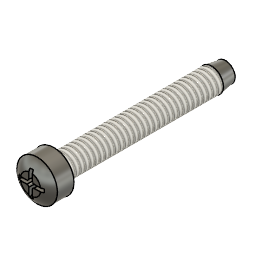
modelo_completo_v3 (Autodesk Fusion 360 archive; units mm, degrees)
design "Tornillo autorroscante taladrado con hueco cruciforme de tipo I ANSI B18.6.4 1/4-20 UNC x 1.75 Tipo C Acero grado 2 Normal"
description: Tornillo autorroscante taladrado con hueco cruciforme de tipo I ANSI B18.6.4 1/4-20 UNC x 1.75 Tipo C
part number: CRFHTSTCTI ANSI B18.6.4 - 1/4 - 20 x 1 3/4 Acero grado 2 Normal
Autodesk Fusion 360 part; units mm, degrees
note: some values were not read from the file. Chosen so that the rebuilt part matches the saved one: which bodies a step acts on; which face or edge a step refers to; how an offset face is resized; the sign of a taper; which pieces of a blend or face edit are solid. Set by a fixed rule: which sketch regions a step uses.
sketch "Sketch1" plane through (0, 0, 0) normal (0, 1, 0) x (1, 0, 0)
  line L0 (-3.175, 0) -> (-3.175, 44.45)
  line L1 (-3.175, 44.45) -> (0, 44.45)
  line L2 (0, 44.45) -> (0, -6.0198)
  line L3 (-3.175, 0) -> (-5.2578, 0)
  line L4 (-5.2578, 0) -> (-5.2578, -4.318)
  arc A0 (-5.2578, -4.318) -> (-2.6289, -6.0198) centre (0, 0.9227) ccw
  line L5 (0, -6.0198) -> (-2.6289, -6.0198)
  dimension "d9" = 6.35
  dimension "d66" = 10.5156
  dimension "d122" = 6.0198
  dimension "d123" = 1.7018
  dimension "d124" = 5.2578
  dimension "d125" = 44.45
  constraint perpendicular L0 L1
  constraint perpendicular L0 L3
  constraint coincident origin L3
  constraint vertical L0
  constraint vertical L2
  constraint coincident L2 A0.centre
  constraint coincident origin L2
  constraint vertical L4
  constraint perpendicular L2 L5
  constraint coincident L2 L5.start
  constraint coincident L2.end L5.start
  measures "d122" distance of L3 L5
  measures "d123" distance of L4.end L5
  measures "d125" distance of origin L1
revolve "Revolve1" add sketch "Sketch1" angle 360 about axis through (0, 0, -44.45) along (0, 0, 1) makes body 1
ref_plane "WorkPlane1" through (0, 0, 6.0198) normal (0, 0, 1) x (1, 0, 0)
sketch "Sketch2" plane through (0, 0, 6.0198) normal (0, 0, 1) x (1, 0, 0)
  line L0 (-0.4572, -0.4572) -> (-3.4798, -0.4572)
  line L1 (-3.4798, 0.4572) -> (-0.4572, 0.4572)
  line L2 (-3.4798, -0.4572) -> (-3.4798, 0.4572)
  line L3 (-0.4572, -3.4798) -> (-0.4572, -0.4572)
  line L4 (0.4572, -3.4798) -> (-0.4572, -3.4798)
  line L5 (0.4572, -0.4572) -> (0.4572, -3.4798)
  line L6 (3.4798, -0.4572) -> (0.4572, -0.4572)
  line L7 (3.4798, 0.4572) -> (3.4798, -0.4572)
  line L8 (0.4572, 0.4572) -> (3.4798, 0.4572)
  line L9 (0.4572, 3.4798) -> (0.4572, 0.4572)
  line L10 (-0.4572, 3.4798) -> (0.4572, 3.4798)
  line L11 (-0.4572, 0.4572) -> (-0.4572, 3.4798)
  circle A0 centre (0, 0) radius 3.4798 construction
  dimension "d132" = 360
  dimension "d138" = 0.9144
  dimension "d139" = 6.9596
  constraint coincident A0.centre origin
  constraint coincident L0.end L2.start
  constraint horizontal L1
  constraint vertical L0.start L1.end
  constraint coincident L1.end L11.start
  constraint perpendicular L1 L2
  constraint tangent L10 A0
  measures "d138" distance of L0 L1
  measures "d139" diameter of A0
extrude "Extrude2" add sketch "Sketch2" against normal blind 3.7592 draft -4 separate body makes body 2
draft "Draft2" angle -30 neutral plane through (0, 0, 6.0198) pull (0, 0, 1) 4 faces at (-3.3922, 0.0648, 4.7667) (0.0648, -3.3922, 4.7667) (3.3922, 0.0648, 4.7667) (0.0648, 3.3922, 4.7667) on bodies 2
fillet "Fillet4" radius 0.4572 4 edges at (-0.3258, 0.3258, 4.1402) (0.3258, 0.3258, 4.1402) (-0.3258, -0.3258, 4.1402) (0.3258, -0.3258, 4.1402) on bodies 2
combine "Combine1" operation cut target body 1 tool bodies 2
thread "Thread1" "ANSI Unified Screw Threads 0.25 1/4-20 UNC 1/4-20 UNC 2A" major diameter 6.2205 minor diameter 4.8108 pitch 1.27 angle 60 resizes the face on face at (-3.1711, 0.1583, -14.8167) on bodies 1
sketch "Sketch5" plane through (0, 0, 0) normal (0, 1, 0) x (1, 0, 0)
  line L0 (-3.2385, 40.005) -> (-2.54, 44.45)
  line L1 (-3.2385, 40.005) -> (-3.2385, 44.45)
  line L2 (0, 44.45) -> (0, -6.0198)
  line L3 (-3.2385, 44.45) -> (0, 44.45)
  dimension "d126" = 0.6985
  dimension "d127" = 3.2385
  dimension "d128" = 4.445
  constraint coincident L2.start L3.end
  constraint perpendicular L2 L3
  constraint coincident L0.end L3
  constraint perpendicular L1 L3
  measures "d126" distance of L0.end L1
  measures "d127" distance of L1 L2.start
  measures "d128" distance of L0.start L3
revolve "Revolve2" cut sketch "Sketch5" angle 360 about axis through (0, 0, -44.45) along (0, 0, 1) bodies 1
equation "d9 = adsk_nomdia"
equation "d66 = adsk_headdia"
equation "d71 = adsk_headh"
equation "adsk_nomlen = 1.75 in"
equation "adsk_headh = 0.237 in"
equation "adsk_headdia = 0.414 in"
equation "adsk_nomdia = 0.25 in"
equation "adsk_phildia = 0.274 in"
equation "adsk_philwidth = 0.036 in"
equation "adsk_phildepth = 0.148 in"
equation "adsk_startlen = 0.175 in"
equation "adsk_endpointdia = 0.20 in"
equation "d111 = -adsk_phildepth"
equation "adsk_ovalh = 0.067 in"
equation "d122 = adsk_headh"
equation "d123 = adsk_ovalh"
equation "d124 = adsk_headdia * 0.5"
equation "d125 = adsk_nomlen"
equation "d126 = ( 0.51 * adsk_nomdia ) - ( adsk_endpointdia / 2 )"
equation "d127 = 0.51 * adsk_nomdia"
equation "d128 = adsk_startlen"
equation "d136 = adsk_philwidth / 2"
equation "d138 = adsk_philwidth"
equation "d139 = adsk_phildia"

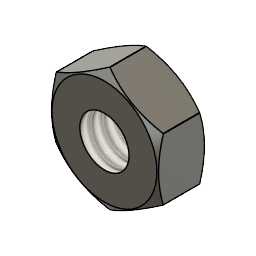
design "Tuerca para maquinaria hexagonal perfil bajo achaflanada ASME B18.6.3 - 1/4-20 Acero grado 2H Normal"
description: Tuerca para maquinaria hexagonal perfil bajo achaflanada ASME B18.6.3 - 1/4-20
part number: CBHMSN ASME B18.6.3 - 1/4-20 Acero grado 2H Normal
Autodesk Fusion 360 part; units mm, degrees
sketch "Sketch1" plane through (0, 0, 0) normal (0, 1, 0) x (1, 0, 0)
  line L0 (0, 0) -> (0, -4.9022)
  line L1 (-3.175, 0) -> (-5.4513, 0)
  line L2 (-5.4513, 0) -> (-6.4135, -0.5555)
  line L3 (-6.4135, -0.5555) -> (-6.4135, -4.3467)
  line L4 (-6.4135, -4.3467) -> (-5.4513, -4.9022)
  line L5 (-5.4513, -4.9022) -> (-3.175, -4.9022)
  line L6 (-3.175, -4.9022) -> (-3.175, 0)
  dimension "d121" = 6.35
  dimension "d122" = 30
  dimension "d123" = 30
  dimension "d128" = 12.827
  dimension "d142" = 10.9027
  dimension "d146" = 4.9022
  constraint vertical L0
  constraint coincident L0 L0.end
  constraint coincident origin L0
  constraint horizontal L1
  constraint coincident L0.start L1
  constraint coincident L0.start origin
  constraint vertical L1.end L4.end
  constraint coincident L0.end L5
  measures "d122" angle of L1 L2
  measures "d123" angle of L4 L5
  measures "d146" distance of L1 L5
revolve "Revolve1" add sketch "Sketch1" angle 360 about axis through (0, 0, 0) along (0, 0, 1)
sketch "Sketch8" plane through (0, 0, 4.9022) normal (0, 0, 1) x (1, 0, 0)
  line L0 (-5.5626, -3.1923) -> (-5.5626, 3.1923)
  circle A0 centre (0, 0) radius 3.175
  circle A1 centre (0, 0) radius 6.4135
  dimension "d114" = 5.5626
  constraint coincident L0.end A1
  constraint coincident L0.start A1
  constraint vertical L0
  measures "d114" distance of A0.centre L0
extrude "Extrude5" cut sketch "Sketch8" against normal blind 4.9022 contours L0 A1 picked at (-5.6999, -0.7773)
pattern_circular "C-Pattern2" count 6 over 360 about axis through (0, 0, 1.75) along (0, 0, 1) of "Extrude5"
thread "Thread3" "ANSI Unified Screw Threads 0.25 1/4-20 UNC 1/4-20 UNC 2B" major diameter 6.35 minor diameter 5.1181 pitch 1.27 angle 60 resizes the face on face at (-3.1711, 0.1583, 3.2681)
equation "d89 = -adsk_nheig"
equation "d114 = adsk_waflat / 2"
equation "adsk_chamang1 = 30 deg"
equation "adsk_chamang2 = 30 deg"
equation "d121 = adsk_nomdia"
equation "d122 = adsk_chamang1"
equation "d123 = adsk_chamang2"
equation "d128 = adsk_maxdia"
equation "adsk_nheig = 0.193 in"
equation "adsk_maxdia = 0.505 in"
equation "adsk_nomdia = 0.25 in"
equation "adsk_waflat = 0.438 in"
equation "d139 = adsk_nheig"
equation "adsk_beardia = adsk_waflat * 0.98"
equation "d142 = adsk_beardia"
equation "d146 = adsk_nheig"

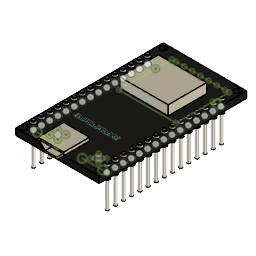
design "PINS"
part number: 2026-06-24-16-48-10-283
Autodesk Fusion 360 part; units mm, degrees
sketch "Boceto1" plane through (0, 0, 0) normal (0, 0, 1) x (1, 0, 0)
  circle A0 centre (-12.7, 17.8) radius 0.5
extrude "Extruir1" add sketch "Boceto1" along normal blind 2.5 and the other way blind 0 makes body 1
sketch "Boceto2" plane through (0, 0, 0) normal (0, 0, 1) x (1, 0, 0)
  line L0 (-14, 24) -> (12, 24)
  line L1 (12, 24) -> (12, -20)
  line L2 (12, -20) -> (-14, -20)
  line L3 (-14, -20) -> (-14, 24)
  constraint horizontal L0
  constraint vertical L1
  constraint horizontal L2
  constraint vertical L3
extrude "Extruir2" add sketch "Boceto2" along normal blind 2 separate body makes body 2
extrude "Extruir3" add 1 faces at (-12.8082, 17.6557, 0) along direction (0, 0, -1) blind 10 on bodies 1 bodies 1 2
extrude "Extruir4" add 1 faces at (3.3333, -20, 0.6667) along direction (0, -1, 0) blind 2 on bodies 1 bodies 1
sketch "Boceto3" plane through (0, 0, 2) normal (0, 0, 1) x (-1, 0, 0)
  line L0 (-12, 22) -> (-12, -24)
  line L1 (-12, -24) -> (14, -24)
  line L2 (14, -24) -> (14, 22)
  line L3 (14, 22) -> (-12, 22)
  circle A0 centre (12.7, -17.8) radius 0.5
  line L4 (12.5, -22.5) -> (12.5, 20.5)
  line L5 (12.5, 20.5) -> (-10.5, 20.5)
  line L6 (-10.5, 20.5) -> (-10.5, -22.5)
  line L7 (-10.5, -22.5) -> (12.5, -22.5)
  dimension "d11" = -1.5
hole "Agujero1" at (-12.5, 22.5, 2) at (10.5, 22.5, 2) at (-12.5, -20.5, 2) at (10.5, -20.5, 2) direction (0, 0, -1) diameter 2 depth 11 tip angle 118 bodies 1
extrude "Extruir5" add 1 faces at (-12.8082, 17.6557, 2.5) along direction (0, 0, 1) blind 0.1 on bodies 1 bodies 1
sketch "Boceto4" plane through (0, 0, 0) normal (0, 0, 1) x (1, 0, 0)
  circle A0 centre (-12.7, 17.8) radius 0.8062
extrude "Extruir6" add sketch "Boceto4" against normal blind 1.5 separate body makes body 3
sketch "Boceto5" plane through (0, 0, 2) normal (0, 0, 1) x (-1, 0, 0)
  circle A0 centre (12.7, -17.8) radius 0.5
  line L0 (-12, 22) -> (-12, -24)
  line L1 (-12, -24) -> (14, -24)
  line L2 (14, -24) -> (14, 22)
  line L3 (14, 22) -> (-12, 22)
  circle A1 centre (-10.5, 20.5) radius 1
  circle A2 centre (-10.5, -22.5) radius 1
  circle A3 centre (12.5, -22.5) radius 1
  circle A4 centre (12.5, 20.5) radius 1
  circle A5 centre (12.7, -17.8) radius 0.8
  constraint concentric A0 A5
extrude "Extruir7" add sketch "Boceto5" along normal blind 0.5 contours A5 bodies 1
extrude "Extruir8" add 1 faces at (-12.8082, 17.6557, 2.6) along direction (0, 0, 1) blind 0.2 on bodies 1 bodies 1
extrude "Extruir9" add 1 faces at (-13.3952, 17.8646, 2.5) along direction (0, 0, 1) blind 0.1 on bodies 1 bodies 1
chamfer "Chaflán1" distance 0.2 distance2 0.6 1 edges at (-11.9541, 18.0893, 2.6) measured on face at (-13.3952, 17.8646, 2.6) on bodies 1
split "Dividir1" by face at (-11.9098, 17.6402, -1) of body 3 bodies 1 makes body 4 at (2.7377, 6.3899, 2)
pattern_linear "Patrón R1" count 15 spacing 2.54 along (0, -1, 0) count 2 spacing 23 along (1, 0, 0) of bodies 1 3 makes body 5 at (-12.2006, 15.2351, -6.6667) makes body 6 at (-12.2006, 12.6951, -6.6667) makes body 7 at (-12.2006, 10.1551, -6.6667) makes body 8 at (-12.2006, 7.6151, -6.6667) makes body 9 at (-12.2006, 5.0751, -6.6667) makes body 10 at (-12.2006, 2.5351, -6.6667) makes body 11 at (-12.2006, -0.0049, -6.6667) makes body 12 at (-12.2006, -2.5449, -6.6667) makes body 13 at (-12.2006, -5.0849, -6.6667) makes body 14 at (-12.2006, -7.6249, -6.6667) makes body 15 at (-12.2006, -10.1649, -6.6667) makes body 16 at (-12.2006, -12.7049, -6.6667) makes body 17 at (-12.2006, -15.2449, -6.6667) makes body 18 at (-12.2302, -17.931, -6.6667) makes body 19 at (10.7698, 17.629, -6.6667) makes body 20 at (10.7994, 15.2351, -6.6667) makes body 21 at (10.7994, 12.6951, -6.6667) makes body 22 at (10.7994, 10.1551, -6.6667) makes body 23 at (10.7994, 7.6151, -6.6667) makes body 24 at (10.7994, 5.0751, -6.6667) makes body 25 at (10.7994, 2.5351, -6.6667) makes body 26 at (10.7994, -0.0049, -6.6667) makes body 27 at (10.7994, -2.5449, -6.6667) makes body 28 at (10.7994, -5.0849, -6.6667) makes body 29 at (10.7994, -7.6249, -6.6667) makes body 30 at (10.7994, -10.1649, -6.6667) makes body 31 at (10.7994, -12.7049, -6.6667) makes body 32 at (10.7994, -15.2449, -6.6667) makes body 33 at (10.7698, -17.931, -6.6667) makes body 34 at (-11.8948, 15.2198, -1) makes body 35 at (-11.8948, 12.6798, -1) makes body 36 at (-11.8948, 10.1398, -1) makes body 37 at (-11.8948, 7.5998, -1) makes body 38 at (-11.8948, 5.0598, -1) makes body 39 at (-11.8948, 2.5198, -1) makes body 40 at (-11.8948, -0.0202, -1) makes body 41 at (-11.8948, -2.5602, -1) makes body 42 at (-11.8948, -5.1002, -1) makes body 43 at (-11.8948, -7.6402, -1) makes body 44 at (-11.8948, -10.1802, -1) makes body 45 at (-11.8948, -12.7202, -1) makes body 46 at (-11.8948, -15.2602, -1) makes body 47 at (-11.9098, -17.9198, -1) makes body 48 at (11.0902, 17.6402, -1) makes body 49 at (11.1052, 15.2198, -1) makes body 50 at (11.1052, 12.6798, -1) makes body 51 at (11.1052, 10.1398, -1) makes body 52 at (11.1052, 7.5998, -1) makes body 53 at (11.1052, 5.0598, -1) makes body 54 at (11.1052, 2.5198, -1) makes body 55 at (11.1052, -0.0202, -1) makes body 56 at (11.1052, -2.5602, -1) makes body 57 at (11.1052, -5.1002, -1) makes body 58 at (11.1052, -7.6402, -1) makes body 59 at (11.1052, -10.1802, -1) makes body 60 at (11.1052, -12.7202, -1) makes body 61 at (11.1052, -15.2602, -1) makes body 62 at (11.0902, -17.9198, -1)
sketch "Boceto6" plane through (0, 0, 2) normal (0, 0, 1) x (-1, 0, 0)
  circle A0 centre (12.7, -17.8) radius 0.8062
  line L0 (-12, 22) -> (-12, -24)
  line L1 (-12, -24) -> (14, -24)
  line L2 (14, -24) -> (14, 22)
  line L3 (14, 22) -> (-12, 22)
  circle A1 centre (-10.5, 20.5) radius 1
  circle A2 centre (-10.5, -22.5) radius 1
  circle A3 centre (12.5, -22.5) radius 1
  circle A4 centre (12.5, 20.5) radius 1
  line L4 (3, 25) -> (-5, 25) construction
  line L5 (-5, 25) -> (-5, 17) construction
  line L6 (-5, 17) -> (3, 17) construction
  line L7 (3, 17) -> (3, 25) construction
  line L8 (3, 25) -> (-5, 17) construction
  line L9 (-5, 25) -> (3, 17) construction
  line L10 (3, 17) -> (-5, 17)
  line L11 (-5, 17) -> (-5, 25)
  line L12 (-5, 25) -> (3, 25)
  line L13 (3, 25) -> (3, 17)
  point P0 (-1, 21)
  dimension "d31" = 8
  dimension "d32" = 8
  constraint horizontal L4
  constraint perpendicular L4 L5
  constraint parallel L4 L6
  constraint parallel L5 L7
  constraint coincident L8 P0
  constraint coincident L9 P0
  constraint horizontal L10
  constraint vertical L11
  constraint horizontal L12
  constraint vertical L13
  measures "d31" distance of L5.end L6.end
  measures "d32" distance of L4.end L5.end
extrude "Extruir10" add sketch "Boceto6" along normal blind 3 separate body contours L3 L11 L12 L13 | L3 L10 L11 L13 makes body 63
chamfer "Chaflán2" distance 2 distance2 2 1 edges at (5, -21, 2) measured on face at (2.3333, -20.3333, 2) on bodies 63
chamfer "Chaflán3" distance 2 distance2 2 1 edges at (-3, -21, 2) measured on face at (-1, -19.6667, 2) on bodies 63
sketch "Boceto7" plane through (0, -25, 0) normal (0, -1, 0) x (1, 0, 0)
  line L0 (-3, 5) -> (-3, 4)
  line L1 (-3, 4) -> (-1, 2)
  line L2 (-1, 2) -> (3, 2)
  line L3 (3, 2) -> (5, 4)
  line L4 (5, 4) -> (5, 5)
  line L5 (5, 5) -> (-3, 5)
  line L6 (-2.5, 4.2071) -> (-0.7929, 2.5)
  line L7 (-0.7929, 2.5) -> (2.7929, 2.5)
  line L8 (2.7929, 2.5) -> (4.5, 4.2071)
  line L9 (4.5, 4.2071) -> (4.5, 4.5)
  line L10 (4.5, 4.5) -> (-2.5, 4.5)
  line L11 (-2.5, 4.5) -> (-2.5, 4.2071)
  dimension "d41" = -0.5
extrude "Extruir12" cut sketch "Boceto7" against normal blind 7 contours L6 L7 L8 L9 L10 L11 bodies 63
move_body "Desplazar1" bodies 63 to x (1, 0, 0) y (0, 1, 0) z (0, 0, 1) at (-1, 0, 0)
sketch "Boceto8" plane through (0, 0, 2) normal (0, 0, 1) x (-1, 0, 0)
  circle A0 centre (12.7, -17.8) radius 0.8062
  line L0 (-12, 22) -> (-12, -24)
  line L1 (-12, -24) -> (14, -24)
  line L2 (14, -24) -> (14, 22)
  line L3 (14, 22) -> (-12, 22)
  circle A1 centre (-10.5, 20.5) radius 1
  circle A2 centre (-10.5, -22.5) radius 1
  circle A3 centre (12.5, -22.5) radius 1
  circle A4 centre (12.5, 20.5) radius 1
  line L4 (1, -24) -> (1, -17)
  line L5 (8.5, -17) -> (-6.5, -17)
  line L6 (8.5, -17) -> (-6.5, -17)
  line L7 (-6.5, -17) -> (-6.5, -5)
  line L8 (-6.5, -5) -> (8.5, -5)
  line L9 (8.5, -5) -> (8.5, -17)
  dimension "d44" = 7
  dimension "d45" = 15
  dimension "d46" = 12
  constraint midpoint L1 L4.start
  constraint perpendicular L1 L4
  constraint horizontal L5
  constraint midpoint L4.end L5
  constraint horizontal L6
  constraint vertical L7
  constraint horizontal L8
  constraint vertical L9
  measures "d44" distance of L4.start L4.end
  measures "d45" distance of L5.start L5.end
  measures "d46" distance of L5.start L8.end
extrude "Extruir13" add sketch "Boceto8" along normal blind 2 separate body contours L5 L6 L7 L8 L9 makes body 64
extrude "Extruir14" cut 1 faces at (-1, 9, 4) along direction (0, 0, -1) blind 1 on bodies 64 bodies 64
extrude "Extruir15" add 1 faces at (-3.5, 9, 3) along direction (0, 0, 1) blind 2 on bodies 64 bodies 64
move_body "Desplazar2" bodies 63 to x (1, 0, 0) y (0, 1, 0) z (0, 0, 1) at (-1, 1, 0)
